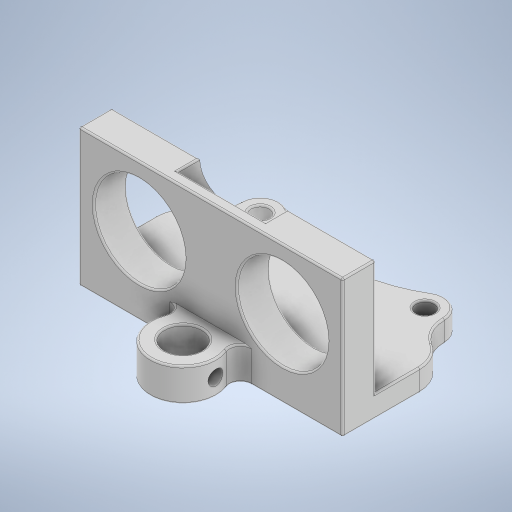
# Autodesk Inventor part: Front Sensor Mount
Saved by Autodesk Inventor 2023 (Build 270158000, 158)
## iProperties
Created: 2023-11-02
Part Number: Front Sensor Mount
Material: Generic
Document SubType Name: Modeling
Designer: Eric
Density: 1 g/cm^3
Appearance: Default
Author: Eric
Autodesk Inventor part; units mm, degrees
ref_plane "YZ Plane" through (0, 0, 0) normal (1, 0, 0) x (0, 1, 0)
ref_plane "XZ Plane" through (0, 0, 0) normal (0, 1, 0) x (-1, 0, 0)
ref_plane "XY Plane" through (0, 0, 0) normal (0, 0, 1) x (1, 0, 0)
sketch "Sketch1" plane through (0, 0, 0) normal (0, 1, 0) x (-1, 0, 0)
  circle A0 centre (15, -5) radius 1.65
  circle A1 centre (-15, -5) radius 1.65
  arc A2 (13.1972, -8) -> (18.5, -5) centre (15, -5) ccw
  arc A3 (-18.5, -5) -> (-13.1972, -8) centre (-15, -5) ccw
  arc A4 (13.1972, -8) -> (-13.1972, -8) centre (0, -29.9615) ccw
  line L0 (24, 5) -> (24, 19)
  line L1 (-24, 5) -> (-24, 19)
  arc A5 (21.25, 0) -> (24, 5) centre (18.0795, 5) ccw
  arc A6 (21.25, 0) -> (18.5, -5) centre (24.4205, -5) ccw
  line L2 (0, -11.9168) -> (0, 19.826) construction
  arc A7 (-24, 5) -> (-21.25, 0) centre (-18.0795, 5) ccw
  arc A8 (-18.5, -5) -> (-21.25, 0) centre (-24.4205, -5) ccw
  circle A9 centre (0, 24) radius 3.4
  arc A10 (5.5621, 21.75) -> (-5.5621, 21.75) centre (0, 24) ccw
  line L3 (24, 19) -> (7.4162, 19)
  line L4 (-7.4162, 19) -> (-24, 19)
  arc A11 (5.5621, 21.75) -> (7.4162, 19) centre (7.4162, 21) ccw
  arc A12 (-7.4162, 19) -> (-5.5621, 21.75) centre (-7.4162, 21) ccw
  point P0 (0, 0)
  point P1 (0, 13)
  point P2 (3.3166, 19)
  point P3 (-3.3166, 19)
  dimension "d0" = 3.3
  dimension "d1" = 30
  dimension "d3" = 3.5
  dimension "d6" = 5
  dimension "d8" = 3
  dimension "d10" = 24
  dimension "d11" = 14
  dimension "d12" = 6.8
  dimension "d14" = 6
  dimension "d15" = 48
  dimension "d16" = 5
  dimension "d17" = 2
  constraints: 22 point on circle, 13 centre point, 12 end point, 9 tangent, 4 equal radius, 4 horizontal alignment, 4 symmetric about line, 3 concentric, 3 point on line, 3 vertical, 2 horizontal, 2 vertical alignment, 1 collinear, 2 other
  measures "d0" diameter of A0
  measures "d1" distance of A1.centre A0.centre
  measures "d3" radius of A2
  measures "d6" vertical distance of point (0, 0) A0.centre
  measures "d8" vertical distance of A0.centre A2.start
  measures "d10" vertical distance of A0.centre L0.end
  measures "d11" distance of L0.start L0.end
  measures "d12" diameter of A9
  measures "d14" radius of A10
  measures "d15" distance between parallel lines of L1 L0
  measures "d16" distance from line of L4 A9.centre
  measures "d17" radius of A11
extrude "Extrusion1" add sketch "Sketch1" along normal blind 4
sketch "Sketch3" plane through (0, 4, 0) normal (0, 1, 0) x (1, 0, 0)
  line L0 (-24, -19) -> (-7.4162, -19) projected
  line L1 (24, -19) -> (24, -5) projected
  line L2 (-24, -19) -> (24, -19)
  line L3 (24, -19) -> (24, -13)
  line L4 (24, -13) -> (-24, -13)
  line L5 (-24, -13) -> (-24, -19)
  point P0 (0, 0)
  point P1 (-7.4162, -19)
  dimension "d23" = 6
  constraints: 8 end point, 2 parallel, 1 horizontal, 1 perpendicular, 1 point on line
  measures "d23" distance between parallel lines of L2 L4
extrude "Extrusion3" add sketch "Sketch3" along normal blind 21
sketch "Sketch4" plane through (7.4162, 0, 19) normal (0, 0, 1) x (1, 0, 0)
  circle A0 centre (-20.4162, 14) radius 8.25
  circle A1 centre (5.5838, 14) radius 8.25
  line L0 (-1.4162, 0) -> (-13.4162, 0) projected
  line L1 (-1.4162, 4) -> (-13.4162, 4) projected
  point P0 (-7.4162, 0)
  point P1 (-12.9783, 0)
  point P2 (-1.854, 0)
  point P3 (-7.4162, 0)
  point P4 (-12.9783, 4)
  point P5 (-1.854, 4)
  dimension "d26" = 26
  dimension "d27" = 16.5
  dimension "d28" = 13
  dimension "d29" = 10
  constraints: 2 centre point, 1 equal radius, 1 horizontal alignment, 1 midpoint
  measures "d26" distance of A1.centre A0.centre
  measures "d27" diameter of A1
  measures "d28" horizontal distance of point (-7.416, 0) A1.centre
  measures "d29" distance from line of L1 A1.centre
extrude "Extrusion4" cut sketch "Sketch4" against normal up to surface (6 mm away)
sketch "Sketch5" plane through (24, 4, 13) normal (0, 0, -1) x (-1, 0, 0)
  line L0 (18.25, 2.75) -> (29.75, 2.75) construction
  line L1 (20.75, 0.25) -> (27.25, 0.25)
  line L2 (27.25, 5.25) -> (20.75, 5.25)
  arc A0 (20.75, 5.25) -> (20.75, 0.25) centre (20.75, 2.75) ccw
  arc A1 (27.25, 0.25) -> (27.25, 5.25) centre (27.25, 2.75) ccw
  circle A2 centre (37, 10) radius 8.25 projected
  line L3 (48, 0) -> (0, 0) projected
  point P0 (24, -4)
  point P1 (24, 2.75)
  point P2 (24, 0)
  dimension "d32" = 11.5
  dimension "d33" = 5
  dimension "d34" = 9.75
  constraints: 8 end point, 7 point on circle, 4 tangent, 2 centre point, 2 midpoint, 2 point on line, 1 horizontal, 1 parallel, 1 vertical alignment
  measures "d32" distance of point (18.25, 2.75) L0.end
  measures "d33" distance between parallel lines of L1 L2
  measures "d34" distance from line of A2.centre L1
extrude "Extrusion5" cut sketch "Sketch5" against normal blind 4 contours A0 L2 A1 L1
sketch "Sketch6" plane through (24, 4, 13) normal (0, 0, -1) x (-1, 0, 0)
  line L0 (48, 21) -> (0, 21) projected
  line L1 (16, 21) -> (32, 21) construction
  line L2 (20.5, 25.5) -> (27.5, 25.5)
  line L3 (27.5, 16.5) -> (20.5, 16.5)
  arc A0 (20.5, 25.5) -> (20.5, 16.5) centre (20.5, 21) ccw
  arc A1 (27.5, 16.5) -> (27.5, 25.5) centre (27.5, 21) ccw
  line L4 (20.75, 5.25) -> (27.25, 5.25) projected
  point P0 (24, -4)
  point P1 (24, 21)
  point P2 (24, 5.25)
  point P3 (24, 5.25)
  point P4 (32, 21)
  point P5 (16, 21)
  dimension "d37" = 16
  dimension "d38" = 9
  constraints: 8 end point, 8 point on circle, 4 point on line, 4 tangent, 3 midpoint, 2 centre point, 1 parallel, 1 vertical alignment
  measures "d37" distance of point (16, 21) point (32, 21)
  measures "d38" distance between parallel lines of L2 L3
extrude "Extrusion6" cut sketch "Sketch6" against normal blind 4 contours A1 L3 A0 L0
sketch "Sketch7" plane through (0, 4, 0) normal (0, 1, 0) x (1, 0, 0)
  line L0 (7.4162, -19) -> (-7.4162, -19) projected
  arc A0 (7.4162, -19) -> (5.5621, -21.75) centre (7.4162, -21) ccw projected
  arc A1 (-5.5621, -21.75) -> (5.5621, -21.75) centre (0, -24) ccw projected
  arc A2 (-5.5621, -21.75) -> (-7.4162, -19) centre (-7.4162, -21) ccw projected
  circle A3 centre (0, -24) radius 3.4 projected
  point P0 (0, 0)
extrude "Extrusion7" add sketch "Sketch7" along normal blind 2
sketch "Sketch8" plane through (24, 0, 19) normal (1, 0, 0) x (0, 0, -1)
  line L0 (-8.4, 6) -> (-1.6, 6) projected
  circle A0 centre (-5, 3) radius 1.35
  point P0 (19, 0)
  point P1 (-5, 6)
  dimension "d43" = 2.7
  dimension "d44" = 3
  constraints: 1 centre point, 1 midpoint, 1 vertical alignment
  measures "d43" diameter of A0
  measures "d44" distance from line of L0 A0.centre
extrude "Extrusion8" cut sketch "Sketch8" against normal blind 24
fillet "Fillet1" radius 0.3 52 edges at (-24, 14.5, 13) (-24, 12.5, 19) (24, 12.5, 19) (24, 14.5, 13) (0, 25, 19) (24, 25, 16) (-24, 25, 16) (-16, 25, 13) (-8, 25, 15) (8, 25, 15) (16, 25, 13) (0, 25, 17) (0, 4.25, 13) (5.75, 6.75, 13) (0, 9.25, 13) (-5.75, 6.75, 13) (-21.25, 14, 13) (4.75, 14, 13) (4.75, 14, 19) (-21.25, 14, 19) (-3.4, 6, 24) (5.7579, 6, 19.882) (-5.7579, 6, 19.882) (0, 6, 30) (5.7579, 0, 19.882) (15.7081, 0, 19) (-5.7579, 0, 19.882) (-15.7081, 0, 19) (0, 0, 30) (3.4, 0, 24) (-16.7234, 4, -8.0463) (-19.2329, 4, -2.1468) (-23.2671, 4, 2.1468) (-24, 4, 9) (16.7234, 4, -8.0463) (19.2329, 4, -2.1468) (23.2671, 4, 2.1468) (24, 4, 9) (0, 4, -4.3397) (-16.7234, 0, -8.0463) (-19.2329, 0, -2.1468) (-23.2671, 0, 2.1468) (-24, 0, 12) (16.7234, 0, -8.0463) (19.2329, 0, -2.1468) (23.2671, 0, 2.1468) (24, 0, 12) (0, 0, -4.3397) (-13.35, 4, -5) (-13.35, 0, -5) (16.65, 4, -5) (16.65, 0, -5)
body "Solid1"
